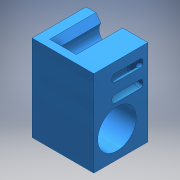
# Autodesk Inventor part: XY h2
Saved by Autodesk Inventor 2016 SP1 (Build 200210100, 210)
## iProperties
Created: 2015-11-19
Part Number: XY h2
Material: Generic
Document SubType Name: Modeling
Designer: PowerStation9000
Density: 1 g/cm^3
Appearance: Cyan
Author: PowerStation9000
Autodesk Inventor part; units mm, degrees
ref_plane "YZ Plane" through (0, 0, 0) normal (1, 0, 0) x (0, 1, 0)
ref_plane "XZ Plane" through (0, 0, 0) normal (0, 1, 0) x (-1, 0, 0)
ref_plane "XY Plane" through (0, 0, 0) normal (0, 0, 1) x (1, 0, 0)
sketch "Sketch1" plane through (0, 0, 0) normal (0, 0, 1) x (1, 0, 0)
  line L0 (-12, 10.5) -> (12, 10.5)
  line L1 (12, 10.5) -> (12, -10.5)
  line L2 (12, -10.5) -> (-12, -10.5)
  line L3 (-12, -10.5) -> (-12, 10.5)
  point P0 (0, 0)
  dimension "d0" = 24
  dimension "d1" = 12
  dimension "d2" = 21
  dimension "d3" = 10.5
  constraints: 8 end point, 2 parallel, 1 horizontal, 1 perpendicular
  measures "d0" distance of L1.end L2.end
  measures "d1" distance from line of point (0, 0) L1
  measures "d2" distance between parallel lines of L0 L2
  measures "d3" distance from line of point (0, 0) L0
extrude "Blok" add sketch "Sketch1" along normal blind 33.5
sketch "Sketch2" plane through (12, -10.5, 0) normal (1, 0, 0) x (0, 0, -1)
  line L0 (0, 0) -> (-33.5, 0) projected
  line L1 (-28.5, 0) -> (-28.5, 21) construction
  line L2 (0, 21) -> (-33.5, 21) projected
  circle A0 centre (-10.5, 9) radius 7.5
  line L3 (0, 21) -> (0, 0) projected
  line L4 (-32.5, 21) -> (-32.5, 0) construction
  line L5 (-24.5, 21) -> (-24.5, 0) construction
  line L6 (0, 0) -> (-33.5, 0) projected
  line L7 (-33.5, 0) -> (-33.5, 21) projected
  point P0 (0, 10.5)
  dimension "d6" = 15
  dimension "d7" = 18
  dimension "d8" = 10.5
  dimension "d9" = 12
  dimension "d11" = 4
  dimension "d12" = 4
  dimension "d13" = 1
  constraints: 6 end point, 6 point on line, 2 vertical, 1 centre point, 1 perpendicular
  measures "d6" diameter of A0
  measures "d7" distance from line of L1 A0.centre
  measures "d8" distance from line of L3 A0.centre
  measures "d9" distance from line of L2 A0.centre
  measures "d11" distance between parallel lines of L1 L4
  measures "d12" distance between parallel lines of L1 L5
  measures "d13" distance between parallel lines of L7 L4
extrude "Lejehul" cut sketch "Sketch2" against normal up to surface (24 mm away) contours A0
sketch "Sketch3" plane through (-12, 10.5, 0) normal (0, 1, 0) x (1, 0, 0)
  line L0 (0, -18) -> (0, -3) construction
  line L1 (24, -3) -> (24, -18) construction
  line L2 (24, 0) -> (24, -33.5) projected
  line L3 (0, -18) -> (24, -18) construction
  line L4 (0, -3) -> (24, -3) construction
  line L5 (0, 0) -> (0, -33.5) projected
  line L6 (0, -3) -> (24, -18) construction
  line L7 (24, -10.5) -> (0, -10.5) construction
  line L8 (24, -28.5) -> (0, -28.5) construction
  arc A0 (18.2766, -30.7943) -> (11.7234, -30.7943) centre (15, -28.5) ccw
  line L9 (11.7234, -30.7943) -> (8.2936, -25.896) construction
  line L10 (18.2766, -30.7943) -> (20.9993, -26.9059) construction
  line L11 (11.7234, -30.7943) -> (18.2766, -30.7943) construction
  line L12 (11.7234, -30.7943) -> (9.8288, -33.5)
  line L13 (18.2766, -30.7943) -> (20.1712, -33.5)
  line L14 (9.8288, -33.5) -> (0, -33.5) construction
  line L15 (20.1712, -33.5) -> (24, -33.5) construction
  line L16 (24, -33.5) -> (24, -33.5)
  line L17 (0, -33.5) -> (0, -33.5)
  line L18 (0, 0) -> (24, 0) projected
  line L19 (24, -33.5) -> (0, -33.5) construction
  line L20 (9.8288, -33.5) -> (20.1712, -33.5)
  line L21 (15, -28.5) -> (15, -33.5)
  point P0 (12, 0)
  point P1 (12, -10.5)
  dimension "d19" = 18
  dimension "d20" = 8
  dimension "d24" = 110
  dimension "d25" = 110
  dimension "d29" = 9
  dimension "d30" = 35
  constraints: 32 end point, 9 point on line, 5 perpendicular, 3 collinear, 3 midpoint, 2 horizontal, 2 parallel, 2 point on circle, 2 tangent, 1 centre point
  measures "d19" distance between parallel lines of L7 L8
  measures "d20" diameter of A0
  measures "d24" angle of L9 L12
  measures "d25" angle of L10 L13
  measures "d29" distance from line of L2 L21.start
  measures "d30" angle of L21 L10
extrude "Tværstang" cut sketch "Sketch3" against normal blind 18
sketch "Sketch4" plane through (12, -10.5, 0) normal (1, 0, 0) x (0, 0, -1)
  line L0 (-29.5, 7) -> (-26.5, 7)
  line L1 (-26.5, 7) -> (-26.5, 19)
  line L2 (-26.5, 19) -> (-29.5, 19)
  line L3 (-29.5, 19) -> (-29.5, 7)
  line L4 (0, 0) -> (-33.5, 0) projected
  line L5 (-33.5, 0) -> (-33.5, 21) projected
  line L6 (-24.5, 2) -> (-24.5, 9) construction
  line L7 (0, 21) -> (-33.5, 21) projected
  point P0 (0, 10.5)
  dimension "d32" = 3
  dimension "d34" = 4
  dimension "d35" = 2
  dimension "d37" = 2
  dimension "d41" = 12
  constraints: 10 end point, 2 parallel, 1 horizontal, 1 perpendicular, 1 vertical
  measures "d32" distance of L1.end L2.end
  measures "d34" distance between parallel lines of L5 L3
  measures "d35" distance between parallel lines of L1 L6
  measures "d37" distance between parallel lines of L7 L2
  measures "d41" distance of L0.end L1.end
revolve "Revolution1" cut sketch "Sketch4" angle 360 about axis through (12, -8.5, 24.5) along (0, 1, 0)
sketch "Sketch5" plane through (-12, -10.5, 0) normal (-1, 0, 0) x (0, 0, 1)
  line L0 (26.5, 7) -> (29.5, 7) projected
  line L1 (26.5, 19) -> (26.5, 7) projected
  line L2 (29.5, 19) -> (26.5, 19) projected
  line L3 (29.5, 7) -> (29.5, 19) projected
  line L4 (24.5, 19) -> (24.5, 12)
  point P0 (0, 10.5)
  dimension "d38" = 2
  constraints: 2 end point, 1 vertical
  measures "d38" distance between parallel lines of L1 L4
revolve "Revolution2" cut sketch "Sketch5" angle 360 about axis through (-12, 8.5, 24.5) along (0, -1, 0)
mirror "Mirror1" about plane through (12, -10.5, 0) normal (1, 0, 0) remove original yes
fillet "Fillet1" radius 1 8 edges at (31, 8.5, 24.5) (34, 8.5, 24.5) (34, -3.5, 24.5) (31, -3.5, 24.5) (17, 8.5, 24.5) (14, 8.5, 24.5) (14, -3.5, 24.5) (17, -3.5, 24.5)
equation "\"d1\" = 0.5 * d0"
equation "\"d3\" = 0.5 * d2"
equation "\"d12\" = d11"
equation "\"d25\" = d24"
body "Solid1"
